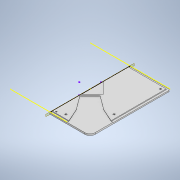
# Autodesk Inventor part: Box_Walls_2
Saved by Autodesk Inventor 2022 (Build 260153000, 153)
## iProperties
Created: 2023-02-27
Part Number: Box_Walls_2
Material: Generic
Document SubType Name: Modeling
Designer: zarek
Density: 1 g/cm^3
Appearance: Default
Author: zarek
Autodesk Inventor part; units mm, degrees
ref_plane "YZ Plane" through (0, 0, 0) normal (1, 0, 0) x (0, 1, 0)
ref_plane "XZ Plane" through (0, 0, 0) normal (0, 1, 0) x (-1, 0, 0)
sketch "Sketch1" plane through (0, 0, 0) normal (0, 1, 0) x (-1, 0, 0)
  line L0 (101.6, -101.6) -> (-101.6, -101.6)
  line L1 (-101.6, -101.6) -> (-101.6, 101.6)
  line L2 (-101.6, 101.6) -> (101.6, 101.6)
  line L3 (101.6, 101.6) -> (101.6, -101.6)
  line L4 (96.6, -96.6) -> (-96.6, -96.6)
  line L5 (-96.6, -96.6) -> (-96.6, 96.6)
  line L6 (-96.6, 96.6) -> (96.6, 96.6)
  line L7 (96.6, 96.6) -> (96.6, -96.6)
  line L8 (101.6, 101.6) -> (-40.4, 101.6)
  circle A0 centre (0, 0) radius 88.9
  circle A1 centre (0, 0) radius 109.3376
  line L9 (-40.4, 101.6) -> (-101.6, 40.4)
  line L10 (-45.4, 101.6) -> (-101.6, 45.4)
  line L11 (96.6, 96.6) -> (96.6, 101.6)
  line L12 (-45.4, 101.6) -> (-35.4, 101.6)
  line L13 (-35.4, 101.6) -> (-35.4, 96.6)
  line L14 (-35.4, 96.6) -> (-45.4, 96.6)
  line L15 (-45.4, 96.6) -> (-45.4, 101.6)
  line L16 (-45.4, 101.6) -> (-43.114, 101.6)
  line L17 (-43.114, 101.6) -> (-43.114, 96.6)
  line L18 (-43.114, 96.6) -> (-45.4, 96.6)
  line L19 (-45.4, 96.6) -> (-45.4, 101.6)
  line L20 (-96.6, 45.4) -> (-101.6, 45.4)
  line L21 (-101.6, 45.4) -> (-101.6, 43.114)
  line L22 (-101.6, 43.114) -> (-96.6, 43.114)
  line L23 (-96.6, 43.114) -> (-96.6, 45.4)
  point P0 (96.6, 51.2168)
  point P1 (101.6, 40.4)
  point P2 (101.6, -40.4)
  point P3 (96.6, -51.2168)
  point P4 (-96.6, 45.4)
  point P5 (-45.4, 96.6)
  dimension "d0" = 203.2
  dimension "d1" = 203.2
  dimension "d2" = 101.6
  dimension "d3" = 101.6
  dimension "d4" = 5
  dimension "d5" = 5
  dimension "d6" = 5
  dimension "d7" = 5
  dimension "d10" = 142
  dimension "d12" = 61.2
  dimension "d14" = 177.8
  dimension "d15" = 5
  dimension "d16" = 5
  dimension "d17" = 10
  dimension "d86" = 2.286
  dimension "d87" = 2.286
  constraints: 48 end point, 11 parallel, 10 point on line, 6 perpendicular, 5 horizontal, 2 centre point, 2 coincident, 2 point on circle
  measures "d0" distance between parallel lines of L2 L0
  measures "d1" distance between parallel lines of L1 L3
  measures "d2" distance from line of L0 point (0, 0)
  measures "d3" distance from line of L1 point (0, 0)
  measures "d4" distance between parallel lines of L4 L0
  measures "d5" distance between parallel lines of L1 L5
  measures "d6" distance between parallel lines of L2 L6
  measures "d7" distance between parallel lines of L3 L7
  measures "d10" distance of L2.end L8.end
  measures "d12" distance from line of L1 L8.end
  measures "d14" diameter of A0
  measures "d15" distance of L10.end L9.end
  measures "d16" distance of L10.start L8.end
  measures "d17" distance of L13.end L14.end
  measures "d86" distance of L17.end L18.end
  measures "d87" distance of L21.end L20.end
extrude "Extrusion1" add sketch "Sketch1" along normal blind 5 contours L0 A1 L4 L7 L3 | L0 A1 L4 | A1 L7 L3 | L0 L1 A1 L5 L4 | A1 L7 L4 | L4 A1 L5 L9 L6 L7 | A1 L7 L11 L2 L3 | L4 L5 A1 | A1 L6 L7 | L1 L9 L22 L5 A1 | L11 L6 A1 L2 | L6 L13 L2 A1 | L1 L22 A1 | A1 L22 L9 | L22 L9 L5 | L6 L17 L9 L2 L13 | L1 L20 A1 L22 | A1 L20 L9 L22 | L20 A1 L10 L5 | L5 L10 L6 L9 | A1 L17 L2 | L9 L17 A1 | L6 L9 L17 | L1 L2 L10 A1 L6 L5 | L10 A1 L20 | L10 A1 L5 | L5 A1 L6 L10 | L15 A1 L17 L9 | L6 L10 A1 L15 | L17 A1 L15 L2 | L5 L6 A1 | L6 A1 L10 | A1 L10 L15 | A0
sketch "Sketch3" plane through (0, 5, 0) normal (0, 1, 0) x (1, 0, 0)
  circle A0 centre (0, 0) radius 88.9
  line L0 (-101.6, 101.6) -> (-101.6, -101.6) projected
  line L1 (-101.6, -101.6) -> (101.6, -101.6) projected
  line L2 (-101.6, 101.6) -> (101.6, 101.6)
  line L3 (101.6, 101.6) -> (101.6, -101.6)
  line L4 (101.6, -101.6) -> (-101.6, -101.6)
  line L5 (-101.6, -101.6) -> (-101.6, 101.6)
  line L6 (-96.6, 96.6) -> (96.6, 96.6)
  line L7 (96.6, 96.6) -> (96.6, -96.6)
  line L8 (96.6, -96.6) -> (-96.6, -96.6)
  line L9 (-96.6, -96.6) -> (-96.6, 96.6)
  line L10 (-101.6, -101.6) -> (40.4, -101.6)
  circle A1 centre (0, 0) radius 109.3376
  line L11 (40.4, -101.6) -> (101.6, -40.4)
  line L12 (101.6, -101.6) -> (101.6, 101.6) projected
  line L13 (45.4038, -101.6) -> (101.6, -45.4038)
  line L14 (96.6, -45.4) -> (101.6, -45.4038)
  line L15 (45.4, -96.6) -> (45.4038, -101.6)
  line L16 (96.6, -45.4) -> (101.6, -45.4)
  line L17 (101.6, -45.4) -> (101.6, -43.114)
  line L18 (101.6, -43.114) -> (96.6, -43.114)
  line L19 (96.6, -43.114) -> (96.6, -45.4)
  line L20 (45.4038, -101.6) -> (43.1178, -101.6)
  line L21 (43.1178, -101.6) -> (43.1178, -96.6)
  line L22 (43.1178, -96.6) -> (45.4038, -96.6)
  line L23 (45.4038, -96.6) -> (45.4038, -101.6)
  point P0 (45.4038, -101.6)
  point P1 (50.4038, -96.6)
  point P2 (96.6, -50.4038)
  dimension "d28" = 177.8
  dimension "d29" = 5
  dimension "d30" = 5
  dimension "d31" = 5
  dimension "d32" = 5
  dimension "d33" = 142
  dimension "d76" = 5.0038
  dimension "d77" = 5.0038
  dimension "d88" = 2.286
  dimension "d89" = 2.286
  constraints: 42 end point, 10 point on line, 9 parallel, 4 horizontal, 4 perpendicular, 2 centre point, 2 coincident, 2 point on circle
  measures "d28" diameter of A0
  measures "d29" distance between parallel lines of L3 L7
  measures "d30" distance between parallel lines of L6 L2
  measures "d31" distance between parallel lines of L0 L9
  measures "d32" distance between parallel lines of L1 L8
  measures "d33" distance of L4.end L10.end
  measures "d76" distance of L13.end L11.end
  measures "d77" distance of L13.start L10.end
  measures "d88" distance of L17.end L16.end
  measures "d89" distance of L21.end L22.end
extrude "Extrusion3" cut sketch "Sketch3" against normal blind 2 contours L2 A1 L6 L9 L0 | A1 L9 L0 | L2 A1 L6 | A1 L9 L8 L1 L0 | L2 L3 A1 L7 L6 | A1 L8 L21 L11 L1 | L3 L11 L18 L7 A1 | A1 L21 L1 | L11 L21 A1 | L3 L18 A1 | A1 L18 L11
sketch "Sketch4" plane through (0, 5, 0) normal (0, 1, 0) x (1, 0, 0)
  line L0 (101.6, 101.6) -> (-101.6, 101.6)
  line L1 (-101.6, 101.6) -> (-101.6, -101.6)
  line L2 (-101.6, -101.6) -> (101.6, -101.6)
  line L3 (101.6, -101.6) -> (101.6, 101.6)
  circle A0 centre (0, 0) radius 2.5
  line L4 (11.3314, 2.139) -> (-2.139, -11.3314)
  line L5 (0, 0) -> (-5.6569, 5.6569)
  line L6 (-5.6569, -14.8492) -> (-26.163, 5.6569)
  line L7 (-5.6569, 26.163) -> (14.8492, 5.6569)
  circle A1 centre (-5.6569, 5.6569) radius 14
  line L8 (-26.163, 5.6569) -> (-5.6569, 26.163)
  line L9 (14.8492, 5.6569) -> (-5.6569, -14.8492)
  line L10 (-40.3051, 5.6569) -> (-5.6569, 40.3051)
  line L11 (-5.6569, 40.3051) -> (28.9914, 5.6569)
  line L12 (28.9914, 5.6569) -> (-5.6569, -28.9914)
  line L13 (-5.6569, -28.9914) -> (-40.3051, 5.6569)
  line L14 (-22.6451, 9.1747) -> (-9.1747, 22.6451)
  line L15 (-9.1747, 22.6451) -> (-12.7668, 26.2372)
  line L16 (-12.7668, 26.2372) -> (-26.2372, 12.7668)
  line L17 (-26.2372, 12.7668) -> (-22.6451, 9.1747)
  point P0 (9.525, 22.5)
  point P1 (-9.525, -6.5)
  dimension "d37" = 203.2
  dimension "d38" = 203.2
  dimension "d39" = 8
  dimension "d40" = 28
  dimension "d41" = 29
  dimension "d42" = 29
  dimension "d43" = 14.5
  dimension "d44" = 10
  dimension "d45" = 10
  dimension "d46" = 10
  dimension "d47" = 10
  dimension "d48" = 5.08
  dimension "d49" = 9.525
  dimension "d50" = 9.525
  dimension "d55" = 101.6
  dimension "d56" = 101.6
  constraints: 36 end point, 8 parallel, 4 perpendicular, 2 centre point, 2 coincident, 2 point on line, 1 horizontal
  measures "d37" distance between parallel lines of L2 L0
  measures "d38" distance between parallel lines of L1 L3
  measures "d39" distance of L5.start L5.end
  measures "d40" diameter of A1
  measures "d41" distance between parallel lines of L9 L8
  measures "d42" distance between parallel lines of L7 L6
  measures "d43" distance from line of A1.centre L8
  measures "d44" distance between parallel lines of L11 L7
  measures "d45" distance between parallel lines of L8 L10
  measures "d46" distance between parallel lines of L13 L6
  measures "d47" distance between parallel lines of L12 L9
  measures "d48" distance between parallel lines of L14 L16
  measures "d49" distance from line of A1.centre L15
  measures "d50" distance from line of L5.end L17
  measures "d55" distance from line of point (0, 0) L1
  measures "d56" distance from line of L0 point (0, 0)
extrude "Extrusion4" cut sketch "Sketch4" against normal blind 1 contours A0 | L4 L9 L6 L8 L7 | L8 L17 L16 L15 | A1 | L10 L11 L12 L13
sketch "Sketch6" plane through (0, 5, 0) normal (0, 1, 0) x (1, 0, 0)
  line L0 (45.4038, -101.6) -> (0, 0)
  line L1 (50.4038, -96.6) -> (45.4038, -101.6) projected
  line L2 (96.6, -43.114) -> (96.6, 96.6) projected
  line L3 (101.6, -101.6) -> (101.6, 101.6) projected
  circle A0 centre (0, 0) radius 34.925
  circle A1 centre (0, 0) radius 33.425
  line L4 (-101.6, 101.6) -> (-101.6, -101.6) projected
  line L5 (-101.6, -101.6) -> (40.4, -101.6)
  line L6 (-101.6, -101.6) -> (101.6, -101.6) projected
  line L7 (101.6, 101.6) -> (101.6, -43.114) projected
  line L8 (101.6, -45.4038) -> (0, 0)
  line L9 (-96.6, -96.6) -> (43.1178, -96.6) projected
  line L10 (96.6, -43.114) -> (96.6, 96.6) projected
  line L11 (43.1178, -101.6) -> (-101.6, -101.6) projected
  line L12 (101.6, -45.4038) -> (96.6, -50.4038) projected
  line L13 (45.4038, -101.6) -> (101.6, -45.4038)
  line L14 (43.1178, -101.6) -> (101.6, -101.6) projected
  line L15 (0, 0) -> (101.6, -50.4076)
  line L16 (50.4076, -101.6) -> (0, 0)
  line L17 (43.1694, -96.6) -> (47.9269, -96.6)
  line L18 (96.6, -43.1694) -> (96.6, -47.9269)
  line L19 (40.4, -101.6) -> (101.6, -40.4)
  point P0 (13.6374, -30.5164)
  point P1 (30.5164, -13.6374)
  point P2 (14.2494, -31.8859)
  point P3 (31.2861, -15.5222)
  point P4 (29.9423, -14.8555)
  point P5 (31.8859, -14.2494)
  point P6 (98.2555, -48.7483)
  point P7 (96.6, -47.9269)
  point P8 (47.9269, -96.6)
  point P9 (15.5222, -31.2861)
  point P10 (96.6, -45.4)
  point P11 (45.4, -96.6)
  point P12 (14.8555, -29.9423)
  point P13 (96.6, -45.4)
  point P14 (45.4, -96.6)
  point P15 (45.4, -96.6)
  point P16 (47.089, -94.911)
  point P17 (94.911, -47.089)
  point P18 (96.6, -45.4)
  point P19 (43.8583, -98.1417)
  point P20 (98.1417, -43.8583)
  point P21 (45.4, -96.6)
  point P22 (96.6, -45.4)
  dimension "d71" = 69.85
  dimension "d72" = 66.85
  dimension "d75" = 142
  dimension "d78" = 5.0038
  dimension "d82" = 5.0038
  constraints: 18 end point, 11 point on line, 2 centre point, 2 coincident, 1 collinear, 1 perpendicular
  measures "d71" diameter of A0
  measures "d72" diameter of A1
  measures "d75" distance of L4.end L5.end
  measures "d78" distance of L0.start L5.end
  measures "d82" distance of L8.start L19.end
extrude "Extrusion6" cut sketch "Sketch6" against normal blind 1 contours L0 A0 L16 L19 L17 | L0 A1 L16 A0 | L16 A1 L15 A0 | L15 A0 L8 L18 L19 | A0 L15 A1 L8
fillet "Fillet3" radius 12.7 1 edges at (101.6, 2.5, 101.6)
sketch "Sketch9" plane through (0, 4, 0) normal (0, 1, 0) x (1, 0, 0)
  point P0 (0, 0)
sketch "Sketch10" plane through (0, 5, 0) normal (0, 1, 0) x (1, 0, 0)
  point P0 (0, 0)
ref_plane "Work Plane1" through (24.6957, 5, 24.6957) normal (0.7071068, 0, 0.7071068) x (0.7071068, 0, -0.7071068)
sketch "Sketch15" plane through (0, 5, 0) normal (0, 1, 0) x (1, 0, 0)
  line L0 (43.1694, -96.6) -> (13.6374, -30.5164) projected
  line L1 (28.4034, -63.5582) -> (-0.6569, -23.9914)
  line L2 (28.9914, 5.6569) -> (-5.6569, -28.9914) projected
  line L3 (30.5164, -13.6374) -> (96.6, -43.1694) projected
  line L4 (-5.6569, 40.3051) -> (28.9914, 5.6569) projected
  line L5 (63.5582, -28.4034) -> (23.9914, 0.6569)
  line L6 (2.3374, -28.0682) -> (28.0682, -2.3374)
  arc A0 (13.6374, -30.5164) -> (30.5164, -13.6374) centre (0, 0) ccw projected
  line L7 (28.4034, -63.5582) -> (13.6374, -30.5164)
  line L8 (63.5582, -28.4034) -> (30.5164, -13.6374)
  arc A1 (13.6374, -30.5164) -> (30.5164, -13.6374) centre (0, 0) ccw
  line L9 (28.6195, -64.3953) -> (1.6303, -28.7753)
  line L10 (1.6303, -28.7753) -> (2.3374, -28.0682)
  dimension "d138" = 5
  dimension "d139" = 5
  dimension "d140" = 5
  dimension "d168" = 1
  constraints: 14 end point, 4 point on line, 3 point on circle, 2 midpoint, 1 centre point, 1 collinear, 1 concentric, 1 parallel
  measures "d138" horizontal distance of L2.end L1.end
  measures "d139" horizontal distance of L2.start L5.end
  measures "d140" distance between parallel lines of L6 L2
  measures "d168" distance of L6.start L9.end
extrude "Extrusion11" cut sketch "Sketch15" against normal blind 1 contours L1 L6 L5 L3 A0 L0
sketch "Sketch16" plane through (0, 4, 0) normal (0, 1, 0) x (1, 0, 0)
  line L0 (2.3374, -28.0682) -> (28.0682, -2.3374) projected
  line L1 (9.4085, -20.9971) -> (12.944, -24.5327)
  line L2 (12.944, -24.5327) -> (24.5327, -12.944)
  line L3 (24.5327, -12.944) -> (20.9971, -9.4085)
  line L4 (12.944, -24.5327) -> (24.5327, -12.944)
  line L5 (24.5327, -12.944) -> (28.5592, -16.9706)
  line L6 (28.5592, -16.9706) -> (16.9706, -28.5592)
  line L7 (16.9706, -28.5592) -> (12.944, -24.5327)
  line L8 (12.944, -24.5327) -> (5.3317, -32.145)
  line L9 (28.4034, -63.5582) -> (2.3374, -28.0682) projected
  line L10 (24.5327, -12.944) -> (32.145, -5.3317)
  line L11 (28.0682, -2.3374) -> (63.5582, -28.4034) projected
  point P0 (0, 0)
  dimension "d144" = 10
  dimension "d145" = 10
  dimension "d146" = 5
  dimension "d152" = 0
  dimension "d153" = 0
  constraints: 18 end point, 6 perpendicular, 6 point on line
  measures "d144" distance of L0.start L1.start
  measures "d145" distance of L0.end L3.end
  measures "d146" distance between parallel lines of L0 L2
  measures "d152" distance between parallel lines of L7 L1
  measures "d153" distance between parallel lines of L5 L3
extrude "Extrusion12" cut sketch "Sketch16" along normal up to surface (1 mm away)
sketch "Sketch20" plane through (0, 5, 0) normal (0, 1, 0) x (1, 0, 0)
  line L0 (47.089, -94.911) -> (45.4, -96.6) projected
  line L1 (47.089, -94.911) -> (94.9376, -47.0624)
  line L2 (94.1649, -47.8351) -> (33.507, -17.7404)
  line L3 (94.911, -47.089) -> (31.2861, -15.5222) projected
  line L4 (15.5222, -31.2861) -> (47.089, -94.911) projected
  line L5 (17.5265, -33.0758) -> (47.8351, -94.1649)
  arc A0 (15.5222, -31.2861) -> (31.2861, -15.5222) centre (0, 0) ccw projected
  line L6 (33.507, -17.7404) -> (31.7193, -16.8534)
  line L7 (17.5265, -33.0758) -> (16.7531, -31.5169)
  arc A1 (16.7531, -31.5169) -> (31.7193, -16.8534) centre (3.7904, -3.3173) ccw
  dimension "d169" = 1
  dimension "d172" = 1
  constraints: 10 end point, 2 point on circle, 2 point on line, 1 centre point, 1 collinear, 1 parallel
  measures "d169" distance between parallel lines of L2 L3
  measures "d172" distance between parallel lines of L5 L4
extrude "Extrusion13" cut sketch "Sketch20" against normal blind 1 contours L4 A0 L3 L1 L2 L6 A1 L7 L5
sketch "Sketch21" plane through (0, 5, 0) normal (0, 1, 0) x (1, 0, 0)
  line L0 (31.7193, -10.1245) -> (13.6778, -27.9949)
  line L1 (47.8351, -94.1649) -> (45.4, -96.6) projected
  line L2 (13.6778, -27.9949) -> (47.8351, -94.1649)
  line L3 (47.8351, -94.1649) -> (43.1178, -96.6)
  line L4 (43.1178, -96.6) -> (43.1178, -101.6) projected
  line L5 (43.1178, -96.6) -> (43.1178, -101.6)
  line L6 (43.1178, -101.6) -> (100.9338, -101.6)
  line L7 (100.9338, -101.6) -> (101.6, -101.6)
  line L8 (101.6, 101.6) -> (101.6, -43.114) projected
  line L9 (101.6, -43.114) -> (101.6, -101.6)
  line L10 (101.6, -88.9) -> (101.6, 101.6) projected
  line L11 (101.6, -43.114) -> (96.6, -43.114)
  line L12 (96.6, -43.114) -> (91.3373, -46.4322)
  line L13 (94.1649, -47.8351) -> (31.7193, -16.8534) projected
  line L14 (91.3373, -46.4322) -> (27.193, -14.6078)
  constraints: 20 end point, 3 collinear, 3 point on line, 2 perpendicular, 1 horizontal
extrude "Extrusion14" cut sketch "Sketch21" against normal blind 1
sketch "Sketch22" plane through (0, 5, 0) normal (0, 1, 0) x (1, 0, 0)
  point P0 (0, 0)
sketch "Sketch25" plane through (0, 5, 0) normal (0, 1, 0) x (1, 0, 0)
  line L0 (-96.6, 96.6) -> (-96.6, -96.6) projected
  line L1 (96.6, 96.6) -> (-96.6, 96.6) projected
  line L2 (-96.6, 96.6) -> (96.6, 96.6)
  line L3 (96.6, -45.4) -> (45.4, -96.6) projected
  line L4 (96.6, 96.6) -> (96.6, -45.4)
  line L5 (96.6, -45.4) -> (45.4, -96.6)
  line L6 (45.4, -96.6) -> (-96.6, -96.6)
  line L7 (-96.6, -96.6) -> (-96.6, 96.6)
  line L8 (-96.6, 96.6) -> (-89.5289, 89.5289)
  circle A0 centre (-89.5289, 89.5289) radius 5
  circle A1 centre (-89.5289, 89.5289) radius 1.5
  line L9 (-89.5289, 84.5289) -> (-96.6, 84.5289)
  line L10 (-89.5289, 89.5289) -> (-89.5289, 84.5289)
  line L11 (-89.5289, 89.5289) -> (-84.5289, 89.5289)
  line L12 (-84.5289, 96.6) -> (-84.5289, 89.5289)
  line L13 (-96.6, -96.6) -> (-89.5289, -89.5289)
  line L14 (-96.6, -96.6) -> (-86.6, -96.6) construction
  circle A2 centre (-89.5289, -89.5289) radius 5
  circle A3 centre (-89.5289, -89.5289) radius 1.75
  line L15 (-89.5289, -89.5289) -> (-84.5289, -89.5289)
  line L16 (-84.5289, -96.6) -> (-84.5289, -89.5289)
  line L17 (-89.5289, -89.5289) -> (-89.5289, -84.5289)
  line L18 (-96.6, -84.5289) -> (-89.5289, -84.5289)
  line L19 (96.6, 96.6) -> (89.5289, 89.5289)
  circle A4 centre (89.5289, 89.5289) radius 5
  circle A5 centre (89.5289, 89.5289) radius 1.75
  line L20 (89.5289, 89.5289) -> (84.5289, 89.5289)
  line L21 (84.5289, 96.6) -> (84.5289, 89.5289)
  line L22 (89.5289, 89.5289) -> (89.5289, 84.5289)
  line L23 (96.6, 84.5289) -> (89.5289, 84.5289)
  line L24 (96.6, -43.114) -> (96.6, 96.6) projected
  line L25 (-96.6, -96.6) -> (43.1178, -96.6) projected
  line L26 (28.9914, 5.6569) -> (-5.6569, -28.9914) projected
  line L27 (25.4, -25.4) -> (101.6, -25.4)
  line L28 (101.6, -88.9) -> (101.6, 101.6) projected
  line L29 (25.4, -25.4) -> (25.4, -101.6)
  line L30 (43.1178, -101.6) -> (-101.6, -101.6) projected
  line L31 (96.6, -25.4) -> (86.6, -25.4)
  circle A6 centre (86.6, -25.4) radius 5
  circle A7 centre (86.6, -25.4) radius 1.75
  line L32 (25.4, -96.6) -> (25.4, -86.6)
  circle A8 centre (25.4, -86.6) radius 5
  circle A9 centre (25.4, -86.6) radius 1.75
  point P0 (0, 0)
  dimension "d203" = 10
  dimension "d205" = 3
  dimension "d206" = 10
  dimension "d207" = 45
  dimension "d208" = 10
  dimension "d209" = 3.5
  dimension "d210" = 10
  dimension "d211" = 10
  dimension "d212" = 3.5
  dimension "d223" = 76.2
  dimension "d224" = 76.2
  dimension "d225" = 10
  dimension "d226" = 10
  dimension "d227" = 3.5
  dimension "d228" = 10
  dimension "d229" = 10
  dimension "d230" = 3.5
  constraints: 50 end point, 14 point on line, 10 centre point, 9 coincident, 9 perpendicular, 6 point on circle, 5 horizontal, 3 parallel, 2 tangent, 1 collinear, 1 equal length, 1 vertical
  measures "d203" distance of L0.start L8.end
  measures "d205" diameter of A1
  measures "d206" distance of L6.end L13.end
  measures "d207" angle of L14 L13
  measures "d208" diameter of A2
  measures "d209" diameter of A3
  measures "d210" distance of L1.start L19.end
  measures "d211" diameter of A4
  measures "d212" diameter of A5
  measures "d223" distance between parallel lines of L28 L29
  measures "d224" distance between parallel lines of L30 L27
  measures "d225" distance of L31.start L31.end
  measures "d226" diameter of A6
  measures "d227" diameter of A7
  measures "d228" distance of L32.start L32.end
  measures "d229" diameter of A8
  measures "d230" diameter of A9
hole "Hole3" at (-89.5289, 5, 89.5289) at (-89.5289, 5, -89.5289) at (89.5289, 5, -89.5289) at (25.4, 5, 86.6) at (86.6, 5, 25.4) direction (0, -1, 0) diameter 2.85 depth 12.7 tip angle 118 countersink diameter 4.445 countersink angle 82 thread size "M3.5x0.6" class "6H" standard "ANSI Metric M Profile"
sketch "Sketch26" plane through (0, 5, 0) normal (0, 1, 0) x (1, 0, 0)
  line L0 (-96.6, -92.6793) -> (-96.6, -59.6793)
  line L1 (-68.6, -92.6793) -> (-96.6, -92.6793)
  line L2 (-96.6, -96.6) -> (43.1178, -96.6) projected
  line L3 (-68.6, -92.6793) -> (-68.6, -96.6)
  line L4 (-68.6, -92.6793) -> (7.4, -92.6793)
  circle A0 centre (-68.6, -92.6793) radius 1.5
  circle A1 centre (7.4, -92.6793) radius 1.5
  line L5 (-101.6, -101.6) -> (-101.6, 101.6) projected
  point P0 (0, 0)
  dimension "d232" = 3.9207
  dimension "d234" = 76
  dimension "d235" = 3
  dimension "d236" = 3
  dimension "d244" = 33
  constraints: 8 end point, 2 centre point, 2 coincident, 2 horizontal, 1 perpendicular, 1 point on line
  measures "d232" distance between parallel lines of L2 L1
  measures "d234" distance of L1.start L4.end
  measures "d235" diameter of A0
  measures "d236" diameter of A1
  measures "d244" distance from line of L5 L1.start
hole "Hole4" at (-68.6, 5, 92.6793) at (7.4, 5, 92.6793) direction (0, -1, 0) diameter 2.85 depth 2.54 tip angle 118 countersink diameter 3.175 countersink angle 82 thread size "M3.5x0.6" class "6H" standard "ANSI Metric M Profile"
sketch "Sketch28" plane through (0, 0, 0) normal (0, -1, 0) x (1, 0, 0)
  circle A0 centre (-6.3815, -33.9493) radius 1.425
  circle A1 centre (-6.3815, -33.9493) radius 1.425
  circle A2 centre (-33.954, -6.3768) radius 1.425
  circle A3 centre (-33.954, -6.3768) radius 1.425
  circle A4 centre (-5.2831, 22.294) radius 1.425
  circle A5 centre (-5.2831, 22.294) radius 1.425
  circle A6 centre (22.2894, -5.2785) radius 1.5113
  circle A7 centre (22.2894, -5.2785) radius 1.5113
  point P0 (0, 0)
  point P1 (0, 0)
  constraints: 8 centre point, 4 coincident
sketch "Sketch29" plane through (0, 5, 0) normal (0, 1, 0) x (1, 0, 0)
  line L0 (-101.6, 101.6) -> (101.6, 101.6) projected
  line L1 (0, 101.6) -> (0, -101.6)
  line L2 (43.1178, -101.6) -> (-101.6, -101.6) projected
  point P0 (0, 0)
  constraints: 2 end point, 1 midpoint, 1 point on line, 1 vertical
ref_plane "Work Plane2" through (0, 5, -101.6) normal (-1, 0, 0) x (0, 0, 1)
fillet "Fillet5" radius 3.175 2 edges at (101.6, 1.5, -101.6) (-101.6, 1.5, -101.6)
sketch "Sketch32" plane through (0, 0, 0) normal (0, -1, 0) x (1, 0, 0)
  line L0 (-96.6, -96.6) -> (96.6, -96.6)
  line L1 (-96.6, 96.6) -> (-96.6, -96.6)
  line L2 (-96.6, -96.6) -> (-96.6, 96.6)
  line L3 (45.4, 96.6) -> (96.6, 45.4)
  line L4 (-96.6, 96.6) -> (45.4, 96.6)
  line L5 (45.4, 96.6) -> (96.6, 45.4)
  line L6 (96.6, 45.4) -> (96.6, -96.6)
  line L7 (96.6, -96.6) -> (-96.6, -96.6)
  line L8 (-96.6, -96.6) -> (-89.5289, -89.5289)
  circle A0 centre (-89.5289, -89.5289) radius 5
  circle A1 centre (-89.5289, -89.5289) radius 1.5
  line L9 (-84.5289, -89.5289) -> (-84.5289, -96.6)
  line L10 (-89.5289, -89.5289) -> (-84.5289, -89.5289)
  line L11 (-89.5289, -89.5289) -> (-89.5289, -84.5289)
  line L12 (-96.6, -84.5289) -> (-89.5289, -84.5289)
  line L13 (96.6, -96.6) -> (89.5289, -89.5289)
  line L14 (96.6, -96.6) -> (96.6, -86.6) construction
  circle A2 centre (89.5289, -89.5289) radius 5
  circle A3 centre (89.5289, -89.5289) radius 1.75
  line L15 (89.5289, -89.5289) -> (89.5289, -84.5289)
  line L16 (96.6, -84.5289) -> (89.5289, -84.5289)
  line L17 (89.5289, -89.5289) -> (84.5289, -89.5289)
  line L18 (84.5289, -96.6) -> (84.5289, -89.5289)
  line L19 (-96.6, 96.6) -> (-89.5289, 89.5289)
  circle A4 centre (-89.5289, 89.5289) radius 5
  circle A5 centre (-89.5289, 89.5289) radius 1.75
  line L20 (-89.5289, 89.5289) -> (-89.5289, 84.5289)
  line L21 (-96.6, 84.5289) -> (-89.5289, 84.5289)
  line L22 (-89.5289, 89.5289) -> (-84.5289, 89.5289)
  line L23 (-84.5289, 96.6) -> (-84.5289, 89.5289)
  line L24 (43.114, 96.6) -> (-96.6, 96.6)
  line L25 (96.6, -96.6) -> (96.6, 43.1178)
  line L26 (-5.6569, 28.9914) -> (28.9914, -5.6569)
  line L27 (25.4, 25.4) -> (25.4, 101.6)
  line L28 (88.9, 101.6) -> (-101.6, 101.6)
  line L29 (25.4, 25.4) -> (101.6, 25.4)
  line L30 (101.6, 43.1178) -> (101.6, -101.6)
  line L31 (25.4, 96.6) -> (25.4, 86.6)
  circle A6 centre (25.4, 86.6) radius 5
  circle A7 centre (25.4, 86.6) radius 1.75
  line L32 (96.6, 25.4) -> (86.6, 25.4)
  circle A8 centre (86.6, 25.4) radius 5
  circle A9 centre (86.6, 25.4) radius 1.75
  point P0 (0, 0)
  point P1 (0, 0)
  dimension "d251" = 10
  dimension "d252" = 3
  dimension "d253" = 10
  dimension "d254" = 45
  dimension "d255" = 10
  dimension "d256" = 3.5
  dimension "d257" = 10
  dimension "d258" = 10
  dimension "d259" = 3.5
  dimension "d260" = 76.2
  dimension "d261" = 76.2
  dimension "d262" = 10
  dimension "d263" = 10
  dimension "d264" = 3.5
  dimension "d265" = 10
  dimension "d266" = 10
  dimension "d267" = 3.5
  constraints: 66 end point, 14 point on line, 10 centre point, 9 coincident, 9 perpendicular, 6 point on circle, 3 parallel, 2 tangent, 1 collinear, 1 equal length
  measures "d251" distance of L0.start L8.end
  measures "d252" diameter of A1
  measures "d253" distance of L6.end L13.end
  measures "d254" angle of L14 L13
  measures "d255" diameter of A2
  measures "d256" diameter of A3
  measures "d257" distance of L1.start L19.end
  measures "d258" diameter of A4
  measures "d259" diameter of A5
  measures "d260" distance between parallel lines of L28 L29
  measures "d261" distance between parallel lines of L30 L27
  measures "d262" distance of L31.start L31.end
  measures "d263" diameter of A6
  measures "d264" diameter of A7
  measures "d265" distance of L32.start L32.end
  measures "d266" diameter of A8
  measures "d267" diameter of A9
hole "Hole5" at (25.4, 0, 86.6) at (86.6, 0, 25.4) at (89.5289, 0, -89.5289) at (-89.5289, 0, -89.5289) at (-89.5289, 0, 89.5289) direction (0, 1, 0) diameter 2.85 depth 12.7 tip angle 118 countersink diameter 5.08 countersink angle 82 thread size "M3.5x0.6" class "6H" standard "ANSI Metric M Profile"
sketch "Sketch33" plane through (0, 5, -101.6) normal (-1, 0, 0) x (0, 0, 1)
  line L0 (239.921, 41.6762) -> (-38.9979, 41.6762)
  line L1 (-38.9979, 41.6762) -> (-38.9979, -40.2918)
  line L2 (-38.9979, -40.2918) -> (239.921, -40.2918)
  line L3 (239.921, -40.2918) -> (239.921, 41.6762)
  point P0 (101.6, -5)
  constraints: 8 end point, 2 parallel, 1 horizontal, 1 perpendicular
extrude "Extrusion18" cut sketch "Sketch33" along normal through all
equation "\"d1\" = d0"
equation "\"d2\" = 0.5 * d0"
equation "\"d3\" = 0.5 * d0"
body "Solid1"
